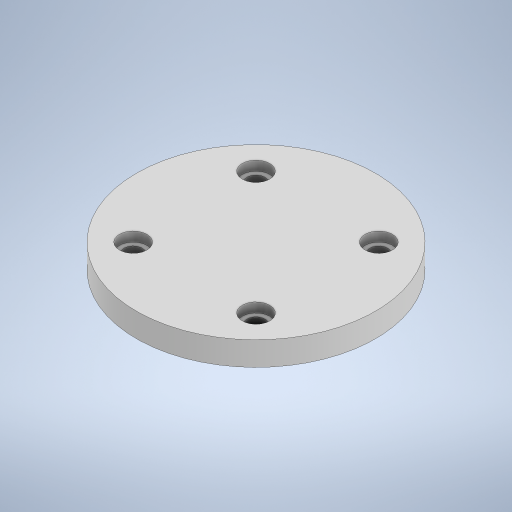
# Autodesk Inventor part: PrismCageAdapter
Saved by Autodesk Inventor 2023 (Build 270158000, 158)
## iProperties
Created: 2024-01-10
Part Number: PrismCageAdapter
Material: Generic
Document SubType Name: Modeling
Designer: kerlin
Density: 1 g/cm^3
Appearance: Default
Author: kerlin
Autodesk Inventor part; units mm, degrees
ref_plane "YZ Plane" through (0, 0, 0) normal (1, 0, 0) x (0, 1, 0)
ref_plane "XZ Plane" through (0, 0, 0) normal (0, 1, 0) x (-1, 0, 0)
ref_plane "XY Plane" through (0, 0, 0) normal (0, 0, 1) x (1, 0, 0)
sketch "Sketch1" plane through (0, 0, 0) normal (0, 1, 0) x (-1, 0, 0)
  circle A0 centre (0, 0) radius 25
  dimension "d0" = 50
  constraints: 1 centre point, 1 coincident
  measures "d0" diameter of A0
extrude "Extrusion1" add sketch "Sketch1" along normal blind 5
sketch "Sketch3" plane through (0, 5, 0) normal (0, 1, 0) x (1, 0, 0)
  point P0 (0, 0)
  point P1 (-12.842, -12.842)
  dimension "d25" = 12.842
  dimension "d26" = 12.842
  measures "d25" horizontal distance of point (0, 0) point (-12.842, -12.842)
  measures "d26" horizontal distance of point (0, 0) point (-12.842, -12.842)
hole "Hole2" at (-12.842, 5, 12.842) direction (0, -1, 0) diameter 3.75 depth 14.944 counterbore diameter 5.75 counterbore depth 2
pattern_circular "Circular Pattern1" count 4 over 360 about axis through (0, -10, 0) along (0, 1, 0) of "Hole2"
body "Solid1"
